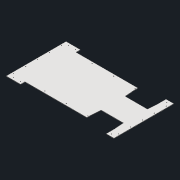
# Autodesk Inventor part: Bellypan
Saved by Autodesk Inventor 2022 (Build 260153000, 153)
## iProperties
Created: 2022-09-10
Part Number: Bellypan
Material: Generic
Document SubType Name: Modeling
Designer: robpl
Density: 1 g/cm^3
Appearance: Default
Author: robpl
Autodesk Inventor part; units mm, degrees
ref_plane "YZ Plane" through (0, 0, 0) normal (1, 0, 0) x (0, 1, 0)
ref_plane "XZ Plane" through (0, 0, 0) normal (0, 1, 0) x (-1, 0, 0)
ref_plane "XY Plane" through (0, 0, 0) normal (0, 0, 1) x (1, 0, 0)
sketch "Sketch2" plane through (0, 0, 0) normal (0, 1, 0) x (-1, 0, 0)
  line L0 (0, 0) -> (-900, 0)
  line L1 (-900, 0) -> (-900, -500)
  line L2 (-900, -500) -> (0, -500)
  line L3 (0, -500) -> (0, 0)
  line L4 (-120, -500) -> (-780, -500)
  line L5 (-780, -500) -> (-780, -463)
  line L6 (-780, -463) -> (-120, -463)
  line L7 (-120, -463) -> (-120, -500)
  line L8 (-120, 0) -> (-780, 0)
  line L9 (-780, 0) -> (-780, -37)
  line L10 (-780, -37) -> (-120, -37)
  line L11 (-120, -37) -> (-120, 0)
  line L12 (-764, -430) -> (-829, -430)
  line L13 (-829, -430) -> (-829, -350)
  line L14 (-829, -350) -> (-764, -350)
  line L15 (-764, -350) -> (-764, -430)
  line L16 (-740, -463) -> (-835, -463)
  line L17 (-835, -463) -> (-835, -430)
  line L18 (-835, -430) -> (-740, -430)
  line L19 (-740, -430) -> (-740, -463)
  line L20 (-740, -430) -> (-764, -350)
  line L21 (-829, -350) -> (-835, -430)
  line L22 (-780, -500) -> (-835, -500)
  line L23 (-835, -500) -> (-835, -463)
  line L24 (-835, -463) -> (-780, -463)
  line L25 (-780, -463) -> (-780, -500)
  line L26 (0, -250) -> (-900, -250)
  line L27 (-829, -150) -> (-764, -150)
  line L28 (-835, -37) -> (-835, -70)
  line L29 (-740, -70) -> (-740, -37)
  line L30 (-740, -70) -> (-764, -150)
  line L31 (-829, -150) -> (-835, -70)
  line L32 (-835, 0) -> (-835, -37)
  point P0 (-780, -463)
  point P1 (-740, -37)
  dimension "d7" = 900
  dimension "d8" = 500
  dimension "d11" = 37
  dimension "d12" = 120
  dimension "d13" = 120
  dimension "d14" = 33
  dimension "d15" = 55
  dimension "d16" = 40
  dimension "d17" = 65
  dimension "d18" = 6
  dimension "d19" = 80
  constraints: 66 end point, 12 parallel, 7 symmetric about line, 6 horizontal, 6 perpendicular, 4 point on line, 2 equal length, 2 midpoint, 1 vertical alignment
  measures "d7" distance of L2.end L1.end
  measures "d8" distance of L1.end L0.end
  measures "d11" distance of L4.end L5.end
  measures "d12" distance between parallel lines of L1 L5
  measures "d13" distance between parallel lines of L3 L7
  measures "d14" distance between parallel lines of L6 L12
  measures "d15" distance between parallel lines of L5 L17
  measures "d16" distance between parallel lines of L5 L19
  measures "d17" distance of L13.end L14.end
  measures "d18" distance between parallel lines of L17 L13
  measures "d19" distance between parallel lines of L12 L14
extrude "Extrusion2" add sketch "Sketch2" along normal blind 3 contours L3 L26 L1 L0 L32 L28 L31 L27 L30 L29 L10 L11 | L3 L2 L7 L6 L19 L20 L14 L21 L17 L23 L1 L26
sketch "Sketch3" plane through (0, 3, 0) normal (0, 1, 0) x (1, 0, 0)
  line L0 (0, 500) -> (0, 0) projected
  line L1 (0, 0) -> (120, 0) projected
  line L2 (120, 500) -> (0, 500) projected
  line L3 (900, 0) -> (900, 500) projected
  point P0 (40, 20)
  point P1 (100, 20)
  point P2 (40, 480)
  point P3 (100, 480)
  point P4 (12.5, 450)
  point P5 (860, 480)
  point P6 (860, 20)
  point P7 (887.5, 450)
  point P8 (12.5, 350)
  point P9 (887.5, 350)
  point P10 (12.5, 250)
  point P11 (887.5, 250)
  point P12 (12.5, 150)
  point P13 (887.5, 150)
  point P14 (12.5, 50)
  point P15 (887.5, 50)
  dimension "d20" = 40
  dimension "d21" = 100
  dimension "d22" = 20
  dimension "d23" = 20
  dimension "d24" = 12.5
  dimension "d25" = 50
  dimension "d33" = 40
  dimension "d34" = 12.5
  dimension "d37" = 100
  dimension "d64" = 50
  constraints: 5 horizontal alignment, 3 vertical alignment, 1 vertical, 8 other
  measures "d20" distance from line of L0 point (40, 20)
  measures "d21" distance from line of L0 point (100, 20)
  measures "d22" distance from line of L1 point (100, 20)
  measures "d23" distance from line of point (40, 480) L2
  measures "d24" distance from line of L0 point (12.5, 450)
  measures "d25" distance from line of L2 point (12.5, 450)
  measures "d33" distance from line of L3 point (860, 20)
  measures "d34" distance from line of L3 point (887.5, 450)
  measures "d37" distance of point (12.5, 450) point (12.5, 350)
  measures "d64" distance from line of L1 point (12.5, 50)
hole "Hole1" at (40, 3, -20) at (100, 3, -20) at (40, 3, -480) at (100, 3, -480) at (12.5, 3, -450) at (860, 3, -480) at (860, 3, -20) at (887.5, 3, -450) at (12.5, 3, -350) at (887.5, 3, -350) at (12.5, 3, -250) at (887.5, 3, -250) at (12.5, 3, -150) at (887.5, 3, -150) at (12.5, 3, -50) at (887.5, 3, -50) direction (0, -1, 0) diameter 5 end through all
sketch "Sketch4" plane through (0, 0, 0) normal (0, -1, 0) x (1, 0, 0)
  line L0 (120, -37) -> (740, -37) projected
  line L1 (740, -463) -> (120, -463) projected
  line L2 (900, 0) -> (900, -500) projected
  point P0 (0, 0)
  point P1 (630, -447.5)
  point P2 (450, -447.5)
  point P3 (270, -447.5)
  point P4 (270, -52.5)
  point P5 (450, -52.5)
  point P6 (630, -52.5)
  dimension "d49" = 15.5
  dimension "d50" = 15.5
  dimension "d51" = 180
  dimension "d52" = 180
  dimension "d53" = 450
  constraints: 4 horizontal alignment, 3 vertical alignment
  measures "d49" distance from line of L0 point (630, -52.5)
  measures "d50" distance from line of L1 point (270, -447.5)
  measures "d51" distance of point (450, -52.5) point (630, -52.5)
  measures "d52" distance of point (270, -52.5) point (450, -52.5)
  measures "d53" distance from line of L2 point (450, -52.5)
hole "Hole2" at (630, 0, -447.5) at (450, 0, -447.5) at (270, 0, -447.5) at (270, 0, -52.5) at (450, 0, -52.5) at (630, 0, -52.5) direction (0, 1, 0) diameter 5 depth 8 tip angle 118
sketch "Sketch5" plane through (0, 0, 0) normal (0, -1, 0) x (1, 0, 0)
  circle A0 centre (450, -52.5) radius 2.5 projected
  circle A1 centre (270, -447.5) radius 2.5 projected
  circle A2 centre (630, -447.5) radius 2.5 projected
  circle A3 centre (450, -447.5) radius 2.5 projected
  circle A4 centre (270, -52.5) radius 2.5 projected
  circle A5 centre (630, -52.5) radius 2.5 projected
  circle A6 centre (12.5, -50) radius 2.5 projected
  circle A7 centre (12.5, -150) radius 2.5 projected
  circle A8 centre (12.5, -250) radius 2.5 projected
  circle A9 centre (12.5, -350) radius 2.5 projected
  circle A10 centre (860, -20) radius 2.5 projected
  circle A11 centre (12.5, -450) radius 2.5 projected
  circle A12 centre (40, -480) radius 2.5 projected
  circle A13 centre (40, -20) radius 2.5 projected
  circle A14 centre (100, -20) radius 2.5 projected
  circle A15 centre (100, -480) radius 2.5 projected
  circle A16 centre (860, -480) radius 2.5 projected
  circle A17 centre (887.5, -450) radius 2.5 projected
  circle A18 centre (887.5, -350) radius 2.5 projected
  circle A19 centre (887.5, -250) radius 2.5 projected
  circle A20 centre (887.5, -150) radius 2.5 projected
  circle A21 centre (887.5, -50) radius 2.5 projected
  line L0 (835, -430) -> (829, -350) projected
  line L1 (835, -500) -> (835, -430) projected
  line L2 (900, -500) -> (835, -500) projected
  line L3 (900, 0) -> (900, -500) projected
  line L4 (835, 0) -> (900, 0) projected
  line L5 (835, -70) -> (835, 0) projected
  line L6 (829, -150) -> (835, -70) projected
  line L7 (764, -150) -> (829, -150) projected
  line L8 (740, -70) -> (764, -150) projected
  line L9 (740, -37) -> (740, -70) projected
  line L10 (120, -37) -> (740, -37) projected
  line L11 (120, 0) -> (120, -37) projected
  line L12 (0, 0) -> (120, 0) projected
  line L13 (0, -500) -> (0, 0) projected
  line L14 (120, -500) -> (0, -500) projected
  line L15 (120, -463) -> (120, -500) projected
  line L16 (740, -463) -> (120, -463) projected
  line L17 (740, -430) -> (740, -463) projected
  line L18 (764, -350) -> (740, -430) projected
  line L19 (829, -350) -> (764, -350) projected
  line L20 (740, -37) -> (740, -70) projected
  line L21 (740, -37) -> (637, -37)
  line L22 (637, -37) -> (637, -70)
  line L23 (637, -70) -> (740, -70)
  line L24 (740, -70) -> (740, -37)
  line L25 (637, -70) -> (643, -150)
  line L26 (829, -150) -> (835, -70) projected
  line L27 (764, -150) -> (829, -150) projected
  line L28 (643, -150) -> (764, -150)
  line L29 (0, -500) -> (0, 0) projected
  line L30 (0, -250) -> (900, -250)
  line L31 (637, -463) -> (637, -430)
  line L32 (637, -430) -> (643, -350)
  line L33 (643, -350) -> (764, -350)
  dimension "d61" = 103
  constraints: 20 end point, 3 symmetric about line, 2 midpoint, 2 parallel, 1 collinear, 1 equal length, 1 horizontal, 1 horizontal alignment, 1 perpendicular
  measures "d61" distance of L8.start L22.end
extrude "Two Motor Cutout" cut sketch "Sketch5" against normal through all contours L31 L32 L33 L18 L17 L16 | L10 L9 L23 L22 | L23 L8 L28 L25
equation "\"d33\" = d20"
equation "\"d34\" = d24"
equation "\"d50\" = d49"
equation "\"d52\" = d51"
body "Solid2"
